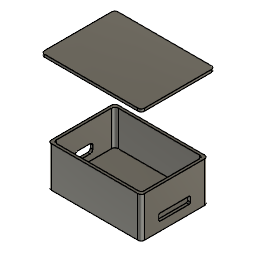
Raspberry Pi Pico Gehäuse Vogelhaus (Autodesk Fusion 360 design; units mm, degrees)
part number: 2026-09-04-17-17-15-442
Autodesk Fusion 360 part; units mm, degrees
note: some values were not read from the file. Set by a fixed rule: which sketch regions a step uses.
sketch "Sketch1" plane through (0, 0, 0) normal (0, 0, 1) x (1, 0, 0)
  line L0 (0, 0) -> (106, 0)
  line L1 (106, 0) -> (106, 76)
  line L2 (106, 76) -> (0, 76)
  line L3 (0, 76) -> (0, 0)
  dimension "d1" = 106
  dimension "d2" = 76
  constraint horizontal L0
  constraint vertical L1
  constraint horizontal L2
  constraint vertical L3
  constraint coincident L0.start L3.end
  measures "d1" distance of L0.start L0.end
  measures "d2" distance of L0.start L2.end
extrude "Extrude1" add sketch "Sketch1" along normal blind 3 makes body 1
extrude "Extrude2" add 1 faces at (35.3333, 50.6667, 3) along direction (0, 0, 1) blind 43 on bodies 1 bodies 1
sketch "Sketch2" plane through (0, 0, 46) normal (0, 0, 1) x (-1, 0, 0)
  line L0 (0, -76) -> (0, 0)
  line L1 (0, 0) -> (-106, 0)
  line L2 (-106, 0) -> (-106, -76)
  line L3 (-106, -76) -> (0, -76)
  line L4 (-3, -73) -> (-3, -3)
  line L5 (-3, -3) -> (-103, -3)
  line L6 (-103, -3) -> (-103, -73)
  line L7 (-103, -73) -> (-3, -73)
  dimension "d7" = -3
extrude "Extrude3" cut sketch "Sketch2" against normal blind 40 contours L4 L5 L6 L7 bodies 1
ref_plane "WorkPlane1" through (53, 38, 126) normal (0, 0, 1) x (1, 0, 0)
sketch "Sketch3" plane through (0, 0, 126) normal (0, 0, 1) x (1, 0, 0)
  line L0 (3, 73) -> (103, 73)
  line L1 (103, 73) -> (103, 3)
  line L2 (103, 3) -> (3, 3)
  line L3 (3, 3) -> (3, 73)
  line L4 (102.85, 3.15) -> (3.15, 3.15)
  line L5 (3.15, 3.15) -> (3.15, 72.85)
  line L6 (3.15, 72.85) -> (102.85, 72.85)
  line L7 (102.85, 72.85) -> (102.85, 3.15)
  point P0 (3, 73)
  point P1 (103, 3)
  dimension "d12" = 0.15
  constraint horizontal L0
  constraint vertical L1
  constraint horizontal L2
  constraint vertical L3
  constraint coincident P1 L1.end
  constraint coincident P0 L0.start
extrude "Extrude4" add sketch "Sketch3" along normal blind 5 separate body contours L4 L5 L6 L7 makes body 2
sketch "Sketch4" plane through (0, 0, 131) normal (0, 0, 1) x (-1, 0, 0)
  line L0 (-102.85, -72.85) -> (-3.15, -72.85)
  line L1 (-3.15, -72.85) -> (-3.15, -3.15)
  line L2 (-3.15, -3.15) -> (-102.85, -3.15)
  line L3 (-102.85, -3.15) -> (-102.85, -72.85)
  line L4 (-109.85, 3.85) -> (-109.85, -79.85)
  line L5 (-109.85, -79.85) -> (3.85, -79.85)
  line L6 (3.85, -79.85) -> (3.85, 3.85)
  line L7 (3.85, 3.85) -> (-109.85, 3.85)
  dimension "d15" = 7
extrude "Extrude5" add sketch "Sketch4" along normal blind 3 contours L0 L1 L2 L3 | L4 L5 L6 L7 bodies 2
sketch "Sketch5" plane through (106, 0, 0) normal (1, 0, 0) x (0, 1, 0)
  line L0 (0, 0) -> (76, 0)
  line L1 (76, 0) -> (76, 46)
  line L2 (76, 46) -> (0, 46)
  line L3 (0, 46) -> (0, 0)
  line L4 (20, 18) -> (56, 18)
  line L5 (56, 18) -> (56, 10)
  line L6 (56, 10) -> (20, 10)
  line L7 (20, 10) -> (20, 18)
  line L8 (38, 10) -> (38, 0)
  dimension "d24" = 8
  dimension "d25" = 36
  dimension "d36" = 10
  constraint horizontal L4
  constraint vertical L5
  constraint horizontal L6
  constraint vertical L7
  constraint midpoint L6 L8.start
  constraint midpoint L0 L8.end
  measures "d24" distance of L4.start L6.end
  measures "d25" distance of L4.start L4.end
  measures "d36" distance of L8.start L8.end
extrude "Extrude6" cut sketch "Sketch5" against normal blind 19 contours L4 L5 L6 L7 bodies 1
sketch "Sketch6" plane through (0, 0, 0) normal (-1, 0, 0) x (0, -1, 0)
  line L0 (-76, 0) -> (0, 0)
  line L1 (0, 0) -> (0, 46)
  line L2 (0, 46) -> (-76, 46)
  line L3 (-76, 46) -> (-76, 0)
  line L4 (-48, 23) -> (-28, 23)
  line L5 (-28, 23) -> (-28, 13)
  line L6 (-28, 13) -> (-48, 13)
  line L7 (-48, 13) -> (-48, 23)
  line L8 (-38, 13) -> (-38, 0)
  dimension "d20" = 20
  dimension "d21" = 10
  dimension "d29" = 13
  constraint horizontal L4
  constraint vertical L5
  constraint horizontal L6
  constraint vertical L7
  constraint midpoint L6 L8.start
  constraint midpoint L0 L8.end
  constraint vertical L8
  measures "d20" distance of L4.start L4.end
  measures "d21" distance of L4.start L6.end
  measures "d29" distance of L8.start L8.end
extrude "Extrude7" cut sketch "Sketch6" against normal blind 30 contours L4 L5 L6 L7 bodies 1
fillet "Fillet1" radius 3 4 edges at (1.5, 48, 23) (1.5, 28, 23) (1.5, 28, 13) (1.5, 48, 13) on bodies 1
fillet "Fillet2" radius 1.5 4 edges at (104.5, 56, 18) (104.5, 56, 10) (104.5, 20, 10) (104.5, 20, 18) on bodies 1
fillet "Fillet3" radius 4 curvature continuous 16 edges at (106, 76, 23) (103, 73, 26) (103, 3, 26) (3, 3, 26) (0, 0, 23) (3, 73, 26) (0, 76, 23) (106, 0, 23) (102.85, 72.85, 128.5) (102.85, 3.15, 128.5) (3.15, 3.15, 128.5) (3.15, 72.85, 128.5) (-3.85, 79.85, 132.5) (109.85, 79.85, 132.5) (109.85, -3.85, 132.5) (-3.85, -3.85, 132.5) on bodies 1 2
